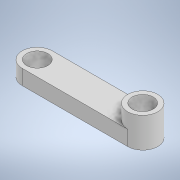
# Autodesk Inventor part: eje de servo 2
Saved by Autodesk Inventor 2021 (Build 250183000, 183)
## iProperties
Created: 2021-03-31
Part Number: eje de servo 2
Material: Generic
Document SubType Name: Modeling
Designer: trejo
Density: 1 g/cm^3
Appearance: Default
Author: trejo
Autodesk Inventor part; units mm, degrees
ref_plane "YZ Plane" through (0, 0, 0) normal (1, 0, 0) x (0, 1, 0)
ref_plane "XZ Plane" through (0, 0, 0) normal (0, 1, 0) x (-1, 0, 0)
ref_plane "XY Plane" through (0, 0, 0) normal (0, 0, 1) x (1, 0, 0)
sketch "Sketch1" plane through (0, 0, 0) normal (0, 1, 0) x (-1, 0, 0)
  line L0 (0, 0) -> (8.75, 0) construction
  circle A0 centre (8.75, 0) radius 1.75
  circle A1 centre (8.75, 0) radius 2.5
  line L1 (0, 0) -> (-8.75, 0) construction
  circle A2 centre (-8.75, 0) radius 1.75
  circle A3 centre (-8.75, 0) radius 2.5
  line L2 (8.75, 2.5) -> (-8.75, 2.5)
  line L3 (8.75, -2.5) -> (-8.75, -2.5)
  dimension "d0" = 8.75
  dimension "d1" = 3.5
  dimension "d2" = 5
  dimension "d3" = 8.75
  dimension "d4" = 3.5
  dimension "d5" = 5
  constraints: 8 end point, 4 centre point, 4 coincident, 4 point on circle, 3 horizontal, 1 tangent
  measures "d0" distance of L0.start L0.end
  measures "d1" diameter of A0
  measures "d2" diameter of A1
  measures "d3" distance of L0.start L1.end
  measures "d4" diameter of A2
  measures "d5" diameter of A3
extrude "Extrusion1" add sketch "Sketch1" along normal blind 2.5
sketch "Sketch2" plane through (0, 2.5, 0) normal (0, 1, 0) x (1, 0, 0)
  circle A0 centre (8.75, 0) radius 1.75 projected
  circle A1 centre (8.75, 0) radius 2.5
  point P0 (0, 0)
  dimension "d8" = 5
  constraints: 1 centre point, 1 coincident
  measures "d8" diameter of A1
extrude "Extrusion2" add sketch "Sketch2" along normal blind 2.5
body "Solid1"
